Autodesk Fusion 360 part; units mm, degrees
(part 7 of 8)
sketch "Sketch4" plane through (0, 0, 10) normal (0, 0, 1) x (-1, 0, 0) in component "Sun Gear"
  arc A0 (-13.3583, 2.9772) -> (-13.4807, 2.3614) centre (0, 0) ccw
  arc A1 (-14.5708, 1.5395) -> (-13.4807, 2.3614) centre (-14.4657, 2.534) ccw
  line L0 (-14.5708, 1.5395) -> (-14.9519, 1.5798)
  spline S0 degree 5 poles (-14.9519, 1.5798) (-14.9606, 1.5807) (-14.978, 1.5823) (-15.0041, 1.5839) (-15.039, 1.5847) (-15.0828, 1.5837) (-15.1266, 1.5812) (-15.1705, 1.578) (-15.2144, 1.5742) (-15.2583, 1.5701) (-15.3023, 1.5657) (-15.3463, 1.5609) (-15.3903, 1.5554) (-15.4343, 1.5493) (-15.4783, 1.5425) (-15.5224, 1.535) (-15.5664, 1.527) (-15.6104, 1.5186) (-15.6545, 1.5097) (-15.6985, 1.5005) (-15.7425, 1.4909) (-15.7866, 1.4808) (-15.8306, 1.4704) (-15.8746, 1.4595) (-15.9186, 1.4482) (-15.9626, 1.4365) (-16.0065, 1.4244) (-16.0505, 1.4119) (-16.0944, 1.3991) (-16.1383, 1.3859) (-16.1822, 1.3724) (-16.2261, 1.3585) (-16.2699, 1.3443) (-16.3137, 1.3297) (-16.3575, 1.3147) (-16.4013, 1.2995) (-16.4451, 1.2839) (-16.4888, 1.2679) (-16.5324, 1.2517) (-16.5761, 1.2351) (-16.6197, 1.2182) (-16.6633, 1.201) (-16.7068, 1.1835) (-16.7504, 1.1657) (-16.7938, 1.1475) (-16.8373, 1.1291) (-16.8807, 1.1104) (-16.924, 1.0913) (-16.9674, 1.072) (-17.0106, 1.0524) (-17.0539, 1.0325) (-17.0971, 1.0123) (-17.1402, 0.9918) (-17.1833, 0.9711) (-17.2264, 0.95) (-17.2694, 0.9287) (-17.3123, 0.9071) (-17.3552, 0.8852) (-17.3981, 0.863) (-17.4409, 0.8406) (-17.4837, 0.8179) (-17.5264, 0.795) (-17.569, 0.7717) (-17.6116, 0.7482) (-17.6541, 0.7245) (-17.6966, 0.7004) (-17.7391, 0.6762) (-17.7814, 0.6516) (-17.8237, 0.6268) (-17.866, 0.6018) (-17.9082, 0.5765) (-17.9419, 0.556) (-17.9671, 0.5405) (-17.9839, 0.5302) (-17.9923, 0.525) knots 0 0 0 0 0 0 0.01428571 0.02857143 0.04285714 0.05714286 0.07142857 0.08571429 0.1 0.11428571 0.12857143 0.14285714 0.15714286 0.17142857 0.18571429 0.2 0.21428571 0.22857143 0.24285714 0.25714286 0.27142857 0.28571429 0.3 0.31428571 0.32857143 0.34285714 0.35714286 0.37142857 0.38571429 0.4 0.41428571 0.42857143 0.44285714 0.45714286 0.47142857 0.48571429 0.5 0.51428571 0.52857143 0.54285714 0.55714286 0.57142857 0.58571429 0.6 0.61428571 0.62857143 0.64285714 0.65714286 0.67142857 0.68571429 0.7 0.71428571 0.72857143 0.74285714 0.75714286 0.77142857 0.78571429 0.8 0.81428571 0.82857143 0.84285714 0.85714286 0.87142857 0.88571429 0.9 0.91428571 0.92857143 0.94285714 0.95714286 0.97142857 0.98571429 1 1 1 1 1 1
  arc A2 (-17.9923, 0.525) -> (-17.9923, -0.525) centre (0, 0) ccw
  spline S1 degree 5 poles (-17.9923, -0.525) (-17.9839, -0.5302) (-17.9671, -0.5405) (-17.9419, -0.556) (-17.9082, -0.5765) (-17.866, -0.6018) (-17.8237, -0.6268) (-17.7814, -0.6516) (-17.7391, -0.6762) (-17.6966, -0.7004) (-17.6541, -0.7245) (-17.6116, -0.7482) (-17.569, -0.7717) (-17.5264, -0.795) (-17.4837, -0.8179) (-17.4409, -0.8406) (-17.3981, -0.863) (-17.3552, -0.8852) (-17.3123, -0.9071) (-17.2694, -0.9287) (-17.2264, -0.95) (-17.1833, -0.9711) (-17.1402, -0.9918) (-17.0971, -1.0123) (-17.0539, -1.0325) (-17.0106, -1.0524) (-16.9674, -1.072) (-16.924, -1.0913) (-16.8807, -1.1104) (-16.8373, -1.1291) (-16.7938, -1.1475) (-16.7504, -1.1657) (-16.7068, -1.1835) (-16.6633, -1.201) (-16.6197, -1.2182) (-16.5761, -1.2351) (-16.5324, -1.2517) (-16.4888, -1.2679) (-16.4451, -1.2839) (-16.4013, -1.2995) (-16.3575, -1.3147) (-16.3137, -1.3297) (-16.2699, -1.3443) (-16.2261, -1.3585) (-16.1822, -1.3724) (-16.1383, -1.3859) (-16.0944, -1.3991) (-16.0505, -1.4119) (-16.0065, -1.4244) (-15.9626, -1.4365) (-15.9186, -1.4482) (-15.8746, -1.4595) (-15.8306, -1.4704) (-15.7866, -1.4808) (-15.7425, -1.4909) (-15.6985, -1.5005) (-15.6545, -1.5097) (-15.6104, -1.5186) (-15.5664, -1.527) (-15.5224, -1.535) (-15.4783, -1.5425) (-15.4343, -1.5493) (-15.3903, -1.5554) (-15.3463, -1.5609) (-15.3023, -1.5657) (-15.2583, -1.5701) (-15.2144, -1.5742) (-15.1705, -1.578) (-15.1266, -1.5812) (-15.0828, -1.5837) (-15.039, -1.5847) (-15.0041, -1.5839) (-14.978, -1.5823) (-14.9606, -1.5807) (-14.9519, -1.5798) knots -1 -1 -1 -1 -1 -1 -0.98571429 -0.97142857 -0.95714286 -0.94285714 -0.92857143 -0.91428571 -0.9 -0.88571429 -0.87142857 -0.85714286 -0.84285714 -0.82857143 -0.81428571 -0.8 -0.78571429 -0.77142857 -0.75714286 -0.74285714 -0.72857143 -0.71428571 -0.7 -0.68571429 -0.67142857 -0.65714286 -0.64285714 -0.62857143 -0.61428571 -0.6 -0.58571429 -0.57142857 -0.55714286 -0.54285714 -0.52857143 -0.51428571 -0.5 -0.48571429 -0.47142857 -0.45714286 -0.44285714 -0.42857143 -0.41428571 -0.4 -0.38571429 -0.37142857 -0.35714286 -0.34285714 -0.32857143 -0.31428571 -0.3 -0.28571429 -0.27142857 -0.25714286 -0.24285714 -0.22857143 -0.21428571 -0.2 -0.18571429 -0.17142857 -0.15714286 -0.14285714 -0.12857143 -0.11428571 -0.1 -0.08571429 -0.07142857 -0.05714286 -0.04285714 -0.02857143 -0.01428571 0 0 0 0 0 0
  line L1 (-14.9519, -1.5798) -> (-14.5708, -1.5395)
  arc A3 (-13.4807, -2.3614) -> (-14.5708, -1.5395) centre (-14.4657, -2.534) ccw
  arc A4 (-13.4807, -2.3614) -> (-13.3583, -2.9772) centre (0, 0) ccw
  arc A5 (-14.0508, -4.1537) -> (-13.3583, -2.9772) centre (-14.3343, -3.1947) ccw
  line L2 (-14.0508, -4.1537) -> (-14.4183, -4.2623)
  spline S2 degree 5 poles (-14.4183, -4.2623) (-14.4267, -4.2648) (-14.4433, -4.27) (-14.4681, -4.2785) (-14.5007, -4.2912) (-14.5407, -4.3088) (-14.5803, -4.3278) (-14.6196, -4.3477) (-14.6587, -4.3679) (-14.6977, -4.3885) (-14.7367, -4.4094) (-14.7754, -4.4307) (-14.814, -4.4526) (-14.8523, -4.4751) (-14.8904, -4.4982) (-14.9282, -4.522) (-14.9658, -4.5462) (-15.0033, -4.5709) (-15.0406, -4.5959) (-15.0777, -4.6213) (-15.1147, -4.647) (-15.1516, -4.6731) (-15.1882, -4.6996) (-15.2247, -4.7265) (-15.2611, -4.7538) (-15.2972, -4.7814) (-15.3332, -4.8094) (-15.369, -4.8378) (-15.4047, -4.8665) (-15.4402, -4.8954) (-15.4756, -4.9247) (-15.5108, -4.9544) (-15.5459, -4.9843) (-15.5808, -5.0145) (-15.6155, -5.0451) (-15.6501, -5.076) (-15.6846, -5.1071) (-15.7188, -5.1386) (-15.753, -5.1703) (-15.787, -5.2023) (-15.8208, -5.2346) (-15.8545, -5.2672) (-15.888, -5.3) (-15.9214, -5.3331) (-15.9546, -5.3665) (-15.9877, -5.4002) (-16.0206, -5.4341) (-16.0534, -5.4683) (-16.086, -5.5027) (-16.1185, -5.5374) (-16.1508, -5.5723) (-16.183, -5.6075) (-16.215, -5.6429) (-16.2469, -5.6786) (-16.2786, -5.7145) (-16.3102, -5.7507) (-16.3416, -5.7871) (-16.3729, -5.8237) (-16.404, -5.8606) (-16.435, -5.8977) (-16.4658, -5.935) (-16.4965, -5.9726) (-16.527, -6.0104) (-16.5573, -6.0484) (-16.5875, -6.0866) (-16.6176, -6.1251) (-16.6475, -6.1637) (-16.6773, -6.2026) (-16.7068, -6.2417) (-16.7363, -6.2811) (-16.7656, -6.3206) (-16.7889, -6.3524) (-16.8063, -6.3763) (-16.8179, -6.3923) (-16.8237, -6.4003) knots 0 0 0 0 0 0 0.01428571 0.02857143 0.04285714 0.05714286 0.07142857 0.08571429 0.1 0.11428571 0.12857143 0.14285714 0.15714286 0.17142857 0.18571429 0.2 0.21428571 0.22857143 0.24285714 0.25714286 0.27142857 0.28571429 0.3 0.31428571 0.32857143 0.34285714 0.35714286 0.37142857 0.38571429 0.4 0.41428571 0.42857143 0.44285714 0.45714286 0.47142857 0.48571429 0.5 0.51428571 0.52857143 0.54285714 0.55714286 0.57142857 0.58571429 0.6 0.61428571 0.62857143 0.64285714 0.65714286 0.67142857 0.68571429 0.7 0.71428571 0.72857143 0.74285714 0.75714286 0.77142857 0.78571429 0.8 0.81428571 0.82857143 0.84285714 0.85714286 0.87142857 0.88571429 0.9 0.91428571 0.92857143 0.94285714 0.95714286 0.97142857 0.98571429 1 1 1 1 1 1
  arc A6 (-16.8237, -6.4003) -> (-16.4218, -7.3704) centre (0, 0) ccw
  spline S3 degree 5 poles (-16.4218, -7.3704) (-16.4121, -7.372) (-16.3926, -7.3751) (-16.3633, -7.3797) (-16.3244, -7.3857) (-16.2757, -7.393) (-16.2271, -7.4) (-16.1785, -7.4067) (-16.13, -7.4131) (-16.0815, -7.4193) (-16.0331, -7.4253) (-15.9847, -7.4309) (-15.9363, -7.4364) (-15.888, -7.4415) (-15.8398, -7.4464) (-15.7916, -7.451) (-15.7435, -7.4553) (-15.6954, -7.4594) (-15.6474, -7.4632) (-15.5994, -7.4667) (-15.5515, -7.4699) (-15.5037, -7.4729) (-15.4559, -7.4756) (-15.4082, -7.478) (-15.3606, -7.4801) (-15.313, -7.482) (-15.2655, -7.4835) (-15.2181, -7.4848) (-15.1708, -7.4858) (-15.1235, -7.4865) (-15.0763, -7.4869) (-15.0292, -7.487) (-14.9822, -7.4868) (-14.9353, -7.4864) (-14.8884, -7.4856) (-14.8417, -7.4845) (-14.795, -7.4831) (-14.7484, -7.4814) (-14.7019, -7.4794) (-14.6555, -7.4771) (-14.6093, -7.4744) (-14.5631, -7.4715) (-14.517, -7.4682) (-14.4711, -7.4645) (-14.4252, -7.4606) (-14.3795, -7.4563) (-14.3339, -7.4517) (-14.2884, -7.4467) (-14.243, -7.4414) (-14.1977, -7.4358) (-14.1526, -7.4298) (-14.1077, -7.4234) (-14.0628, -7.4166) (-14.0182, -7.4094) (-13.9737, -7.4018) (-13.9293, -7.3938) (-13.8851, -7.3855) (-13.841, -7.3768) (-13.7971, -7.3678) (-13.7534, -7.3583) (-13.7098, -7.3484) (-13.6665, -7.3378) (-13.6235, -7.3266) (-13.5808, -7.3148) (-13.5383, -7.3025) (-13.496, -7.2897) (-13.4539, -7.2767) (-13.4118, -7.2633) (-13.3701, -7.2496) (-13.3286, -7.235) (-13.2878, -7.2192) (-13.2559, -7.2052) (-13.2323, -7.1937) (-13.2168, -7.1855) (-13.2092, -7.1813) knots -1 -1 -1 -1 -1 -1 -0.98571429 -0.97142857 -0.95714286 -0.94285714 -0.92857143 -0.91428571 -0.9 -0.88571429 -0.87142857 -0.85714286 -0.84285714 -0.82857143 -0.81428571 -0.8 -0.78571429 -0.77142857 -0.75714286 -0.74285714 -0.72857143 -0.71428571 -0.7 -0.68571429 -0.67142857 -0.65714286 -0.64285714 -0.62857143 -0.61428571 -0.6 -0.58571429 -0.57142857 -0.55714286 -0.54285714 -0.52857143 -0.51428571 -0.5 -0.48571429 -0.47142857 -0.45714286 -0.44285714 -0.42857143 -0.41428571 -0.4 -0.38571429 -0.37142857 -0.35714286 -0.34285714 -0.32857143 -0.31428571 -0.3 -0.28571429 -0.27142857 -0.25714286 -0.24285714 -0.22857143 -0.21428571 -0.2 -0.18571429 -0.17142857 -0.15714286 -0.14285714 -0.12857143 -0.11428571 -0.1 -0.08571429 -0.07142857 -0.05714286 -0.04285714 -0.02857143 -0.01428571 0 0 0 0 0 0
  line L3 (-13.2092, -7.1813) -> (-12.8725, -6.9983)
  arc A7 (-11.5509, -7.3405) -> (-12.8725, -6.9983) centre (-12.3949, -7.8769) ccw
  arc A8 (-11.5509, -7.3405) -> (-11.2021, -7.8625) centre (0, 0) ccw
  arc A9 (-11.3917, -9.2145) -> (-11.2021, -7.8625) centre (-12.0206, -8.437) ccw
  line L4 (-11.3917, -9.2145) -> (-11.6896, -9.4555)
  spline S4 degree 5 poles (-11.6896, -9.4555) (-11.6964, -9.461) (-11.7099, -9.4722) (-11.7295, -9.4895) (-11.7547, -9.5137) (-11.785, -9.5453) (-11.8142, -9.578) (-11.8429, -9.6114) (-11.8713, -9.6451) (-11.8995, -9.679) (-11.9275, -9.7132) (-11.9552, -9.7478) (-11.9824, -9.7827) (-12.0092, -9.8182) (-12.0355, -9.8541) (-12.0614, -9.8905) (-12.0869, -9.9273) (-12.112, -9.9645) (-12.1369, -10.0019) (-12.1615, -10.0395) (-12.1859, -10.0775) (-12.2099, -10.1157) (-12.2336, -10.1542) (-12.2571, -10.193) (-12.2802, -10.2321) (-12.303, -10.2715) (-12.3255, -10.3111) (-12.3478, -10.351) (-12.3698, -10.3911) (-12.3915, -10.4315) (-12.413, -10.4721) (-12.4342, -10.513) (-12.4551, -10.554) (-12.4758, -10.5953) (-12.4962, -10.6369) (-12.5163, -10.6786) (-12.5362, -10.7206) (-12.5559, -10.7628) (-12.5753, -10.8051) (-12.5944, -10.8477) (-12.6133, -10.8905) (-12.632, -10.9335) (-12.6504, -10.9767) (-12.6686, -11.02) (-12.6865, -11.0636) (-12.7042, -11.1074) (-12.7216, -11.1513) (-12.7388, -11.1954) (-12.7558, -11.2397) (-12.7725, -11.2842) (-12.789, -11.3288) (-12.8053, -11.3736) (-12.8213, -11.4186) (-12.8371, -11.4638) (-12.8526, -11.5091) (-12.868, -11.5546) (-12.8831, -11.6003) (-12.8979, -11.6461) (-12.9126, -11.692) (-12.927, -11.7382) (-12.9412, -11.7845) (-12.9551, -11.8309) (-12.9689, -11.8775) (-12.9824, -11.9242) (-12.9956, -11.9711) (-13.0087, -12.0181) (-13.0215, -12.0653) (-13.0341, -12.1126) (-13.0465, -12.16) (-13.0587, -12.2076) (-13.0706, -12.2554) (-13.08, -12.2937) (-13.0869, -12.3224) (-13.0915, -12.3417) (-13.0937, -12.3513) knots 0 0 0 0 0 0 0.01428571 0.02857143 0.04285714 0.05714286 0.07142857 0.08571429 0.1 0.11428571 0.12857143 0.14285714 0.15714286 0.17142857 0.18571429 0.2 0.21428571 0.22857143 0.24285714 0.25714286 0.27142857 0.28571429 0.3 0.31428571 0.32857143 0.34285714 0.35714286 0.37142857 0.38571429 0.4 0.41428571 0.42857143 0.44285714 0.45714286 0.47142857 0.48571429 0.5 0.51428571 0.52857143 0.54285714 0.55714286 0.57142857 0.58571429 0.6 0.61428571 0.62857143 0.64285714 0.65714286 0.67142857 0.68571429 0.7 0.71428571 0.72857143 0.74285714 0.75714286 0.77142857 0.78571429 0.8 0.81428571 0.82857143 0.84285714 0.85714286 0.87142857 0.88571429 0.9 0.91428571 0.92857143 0.94285714 0.95714286 0.97142857 0.98571429 1 1 1 1 1 1
  arc A10 (-13.0937, -12.3513) -> (-12.3513, -13.0937) centre (0, 0) ccw
  spline S5 degree 5 poles (-12.3513, -13.0937) (-12.3417, -13.0915) (-12.3224, -13.0869) (-12.2937, -13.08) (-12.2554, -13.0706) (-12.2076, -13.0587) (-12.16, -13.0465) (-12.1126, -13.0341) (-12.0653, -13.0215) (-12.0181, -13.0087) (-11.9711, -12.9956) (-11.9242, -12.9824) (-11.8775, -12.9689) (-11.8309, -12.9551) (-11.7845, -12.9412) (-11.7382, -12.927) (-11.692, -12.9126) (-11.6461, -12.8979) (-11.6003, -12.8831) (-11.5546, -12.868) (-11.5091, -12.8526) (-11.4638, -12.8371) (-11.4186, -12.8213) (-11.3736, -12.8053) (-11.3288, -12.789) (-11.2842, -12.7725) (-11.2397, -12.7558) (-11.1954, -12.7388) (-11.1513, -12.7216) (-11.1074, -12.7042) (-11.0636, -12.6865) (-11.02, -12.6686) (-10.9767, -12.6504) (-10.9335, -12.632) (-10.8905, -12.6133) (-10.8477, -12.5944) (-10.8051, -12.5753) (-10.7628, -12.5559) (-10.7206, -12.5362) (-10.6786, -12.5163) (-10.6369, -12.4962) (-10.5953, -12.4758) (-10.554, -12.4551) (-10.513, -12.4342) (-10.4721, -12.413) (-10.4315, -12.3915) (-10.3911, -12.3698) (-10.351, -12.3478) (-10.3111, -12.3255) (-10.2715, -12.303) (-10.2321, -12.2802) (-10.193, -12.2571) (-10.1542, -12.2336) (-10.1157, -12.2099) (-10.0775, -12.1859) (-10.0395, -12.1615) (-10.0019, -12.1369) (-9.9645, -12.112) (-9.9273, -12.0869) (-9.8905, -12.0614) (-9.8541, -12.0355) (-9.8182, -12.0092) (-9.7827, -11.9824) (-9.7478, -11.9552) (-9.7132, -11.9275) (-9.679, -11.8995) (-9.6451, -11.8713) (-9.6114, -11.8429) (-9.578, -11.8142) (-9.5453, -11.785) (-9.5137, -11.7547) (-9.4895, -11.7295) (-9.4722, -11.7099) (-9.461, -11.6964) (-9.4555, -11.6896) knots -1 -1 -1 -1 -1 -1 -0.98571429 -0.97142857 -0.95714286 -0.94285714 -0.92857143 -0.91428571 -0.9 -0.88571429 -0.87142857 -0.85714286 -0.84285714 -0.82857143 -0.81428571 -0.8 -0.78571429 -0.77142857 -0.75714286 -0.74285714 -0.72857143 -0.71428571 -0.7 -0.68571429 -0.67142857 -0.65714286 -0.64285714 -0.62857143 -0.61428571 -0.6 -0.58571429 -0.57142857 -0.55714286 -0.54285714 -0.52857143 -0.51428571 -0.5 -0.48571429 -0.47142857 -0.45714286 -0.44285714 -0.42857143 -0.41428571 -0.4 -0.38571429 -0.37142857 -0.35714286 -0.34285714 -0.32857143 -0.31428571 -0.3 -0.28571429 -0.27142857 -0.25714286 -0.24285714 -0.22857143 -0.21428571 -0.2 -0.18571429 -0.17142857 -0.15714286 -0.14285714 -0.12857143 -0.11428571 -0.1 -0.08571429 -0.07142857 -0.05714286 -0.04285714 -0.02857143 -0.01428571 0 0 0 0 0 0
  line L5 (-9.4555, -11.6896) -> (-9.2145, -11.3917)
  arc A11 (-7.8625, -11.2021) -> (-9.2145, -11.3917) centre (-8.437, -12.0206) ccw
  arc A12 (-7.8625, -11.2021) -> (-7.3405, -11.5509) centre (0, 0) ccw
  arc A13 (-6.9983, -12.8725) -> (-7.3405, -11.5509) centre (-7.8769, -12.3949) ccw
  line L6 (-6.9983, -12.8725) -> (-7.1813, -13.2092)
  spline S6 degree 5 poles (-7.1813, -13.2092) (-7.1855, -13.2168) (-7.1937, -13.2323) (-7.2052, -13.2559) (-7.2192, -13.2878) (-7.235, -13.3286) (-7.2496, -13.3701) (-7.2633, -13.4118) (-7.2767, -13.4539) (-7.2897, -13.496) (-7.3025, -13.5383) (-7.3148, -13.5808) (-7.3266, -13.6235) (-7.3378, -13.6665) (-7.3484, -13.7098) (-7.3583, -13.7534) (-7.3678, -13.7971) (-7.3768, -13.841) (-7.3855, -13.8851) (-7.3938, -13.9293) (-7.4018, -13.9737) (-7.4094, -14.0182) (-7.4166, -14.0628) (-7.4234, -14.1077) (-7.4298, -14.1526) (-7.4358, -14.1977) (-7.4414, -14.243) (-7.4467, -14.2884) (-7.4517, -14.3339) (-7.4563, -14.3795) (-7.4606, -14.4252) (-7.4645, -14.4711) (-7.4682, -14.517) (-7.4715, -14.5631) (-7.4744, -14.6093) (-7.4771, -14.6555) (-7.4794, -14.7019) (-7.4814, -14.7484) (-7.4831, -14.795) (-7.4845, -14.8417) (-7.4856, -14.8884) (-7.4864, -14.9353) (-7.4868, -14.9822) (-7.487, -15.0292) (-7.4869, -15.0763) (-7.4865, -15.1235) (-7.4858, -15.1708) (-7.4848, -15.2181) (-7.4835, -15.2655) (-7.482, -15.313) (-7.4801, -15.3606) (-7.478, -15.4082) (-7.4756, -15.4559) (-7.4729, -15.5037) (-7.4699, -15.5515) (-7.4667, -15.5994) (-7.4632, -15.6474) (-7.4594, -15.6954) (-7.4553, -15.7435) (-7.451, -15.7916) (-7.4464, -15.8398) (-7.4415, -15.888) (-7.4364, -15.9363) (-7.4309, -15.9847) (-7.4253, -16.0331) (-7.4193, -16.0815) (-7.4131, -16.13) (-7.4067, -16.1785) (-7.4, -16.2271) (-7.393, -16.2757) (-7.3857, -16.3244) (-7.3797, -16.3633) (-7.3751, -16.3926) (-7.372, -16.4121) (-7.3704, -16.4218) knots 0 0 0 0 0 0 0.01428571 0.02857143 0.04285714 0.05714286 0.07142857 0.08571429 0.1 0.11428571 0.12857143 0.14285714 0.15714286 0.17142857 0.18571429 0.2 0.21428571 0.22857143 0.24285714 0.25714286 0.27142857 0.28571429 0.3 0.31428571 0.32857143 0.34285714 0.35714286 0.37142857 0.38571429 0.4 0.41428571 0.42857143 0.44285714 0.45714286 0.47142857 0.48571429 0.5 0.51428571 0.52857143 0.54285714 0.55714286 0.57142857 0.58571429 0.6 0.61428571 0.62857143 0.64285714 0.65714286 0.67142857 0.68571429 0.7 0.71428571 0.72857143 0.74285714 0.75714286 0.77142857 0.78571429 0.8 0.81428571 0.82857143 0.84285714 0.85714286 0.87142857 0.88571429 0.9 0.91428571 0.92857143 0.94285714 0.95714286 0.97142857 0.98571429 1 1 1 1 1 1
  arc A14 (-7.3704, -16.4218) -> (-6.4003, -16.8237) centre (0, 0) ccw
  spline S7 degree 5 poles (-6.4003, -16.8237) (-6.3923, -16.8179) (-6.3763, -16.8063) (-6.3524, -16.7889) (-6.3206, -16.7656) (-6.2811, -16.7363) (-6.2417, -16.7068) (-6.2026, -16.6773) (-6.1637, -16.6475) (-6.1251, -16.6176) (-6.0866, -16.5875) (-6.0484, -16.5573) (-6.0104, -16.527) (-5.9726, -16.4965) (-5.935, -16.4658) (-5.8977, -16.435) (-5.8606, -16.404) (-5.8237, -16.3729) (-5.7871, -16.3416) (-5.7507, -16.3102) (-5.7145, -16.2786) (-5.6786, -16.2469) (-5.6429, -16.215) (-5.6075, -16.183) (-5.5723, -16.1508) (-5.5374, -16.1185) (-5.5027, -16.086) (-5.4683, -16.0534) (-5.4341, -16.0206) (-5.4002, -15.9877) (-5.3665, -15.9546) (-5.3331, -15.9214) (-5.3, -15.888) (-5.2672, -15.8545) (-5.2346, -15.8208) (-5.2023, -15.787) (-5.1703, -15.753) (-5.1386, -15.7188) (-5.1071, -15.6846) (-5.076, -15.6501) (-5.0451, -15.6155) (-5.0145, -15.5808) (-4.9843, -15.5459) (-4.9544, -15.5108) (-4.9247, -15.4756) (-4.8954, -15.4402) (-4.8665, -15.4047) (-4.8378, -15.369) (-4.8094, -15.3332) (-4.7814, -15.2972) (-4.7538, -15.2611) (-4.7265, -15.2247) (-4.6996, -15.1882) (-4.6731, -15.1516) (-4.647, -15.1147) (-4.6213, -15.0777) (-4.5959, -15.0406) (-4.5709, -15.0033) (-4.5462, -14.9658) (-4.522, -14.9282) (-4.4982, -14.8904) (-4.4751, -14.8523) (-4.4526, -14.814) (-4.4307, -14.7754) (-4.4094, -14.7367) (-4.3885, -14.6977) (-4.3679, -14.6587) (-4.3477, -14.6196) (-4.3278, -14.5803) (-4.3088, -14.5407) (-4.2912, -14.5007) (-4.2785, -14.4681) (-4.27, -14.4433) (-4.2648, -14.4267) (-4.2623, -14.4183) knots -1 -1 -1 -1 -1 -1 -0.98571429 -0.97142857 -0.95714286 -0.94285714 -0.92857143 -0.91428571 -0.9 -0.88571429 -0.87142857 -0.85714286 -0.84285714 -0.82857143 -0.81428571 -0.8 -0.78571429 -0.77142857 -0.75714286 -0.74285714 -0.72857143 -0.71428571 -0.7 -0.68571429 -0.67142857 -0.65714286 -0.64285714 -0.62857143 -0.61428571 -0.6 -0.58571429 -0.57142857 -0.55714286 -0.54285714 -0.52857143 -0.51428571 -0.5 -0.48571429 -0.47142857 -0.45714286 -0.44285714 -0.42857143 -0.41428571 -0.4 -0.38571429 -0.37142857 -0.35714286 -0.34285714 -0.32857143 -0.31428571 -0.3 -0.28571429 -0.27142857 -0.25714286 -0.24285714 -0.22857143 -0.21428571 -0.2 -0.18571429 -0.17142857 -0.15714286 -0.14285714 -0.12857143 -0.11428571 -0.1 -0.08571429 -0.07142857 -0.05714286 -0.04285714 -0.02857143 -0.01428571 0 0 0 0 0 0
  line L7 (-4.2623, -14.4183) -> (-4.1537, -14.0508)
  arc A15 (-2.9772, -13.3583) -> (-4.1537, -14.0508) centre (-3.1947, -14.3343) ccw
  arc A16 (-2.9772, -13.3583) -> (-2.3614, -13.4807) centre (0, 0) ccw
  arc A17 (-1.5395, -14.5708) -> (-2.3614, -13.4807) centre (-2.534, -14.4657) ccw
  line L8 (-1.5395, -14.5708) -> (-1.5798, -14.9519)
  spline S8 degree 5 poles (-1.5798, -14.9519) (-1.5807, -14.9606) (-1.5823, -14.978) (-1.5839, -15.0041) (-1.5847, -15.039) (-1.5837, -15.0828) (-1.5812, -15.1266) (-1.578, -15.1705) (-1.5742, -15.2144) (-1.5701, -15.2583) (-1.5657, -15.3023) (-1.5609, -15.3463) (-1.5554, -15.3903) (-1.5493, -15.4343) (-1.5425, -15.4783) (-1.535, -15.5224) (-1.527, -15.5664) (-1.5186, -15.6104) (-1.5097, -15.6545) (-1.5005, -15.6985) (-1.4909, -15.7425) (-1.4808, -15.7866) (-1.4704, -15.8306) (-1.4595, -15.8746) (-1.4482, -15.9186) (-1.4365, -15.9626) (-1.4244, -16.0065) (-1.4119, -16.0505) (-1.3991, -16.0944) (-1.3859, -16.1383) (-1.3724, -16.1822) (-1.3585, -16.2261) (-1.3443, -16.2699) (-1.3297, -16.3137) (-1.3147, -16.3575) (-1.2995, -16.4013) (-1.2839, -16.4451) (-1.2679, -16.4888) (-1.2517, -16.5324) (-1.2351, -16.5761) (-1.2182, -16.6197) (-1.201, -16.6633) (-1.1835, -16.7068) (-1.1657, -16.7504) (-1.1475, -16.7938) (-1.1291, -16.8373) (-1.1104, -16.8807) (-1.0913, -16.924) (-1.072, -16.9674) (-1.0524, -17.0106) (-1.0325, -17.0539) (-1.0123, -17.0971) (-0.9918, -17.1402) (-0.9711, -17.1833) (-0.95, -17.2264) (-0.9287, -17.2694) (-0.9071, -17.3123) (-0.8852, -17.3552) (-0.863, -17.3981) (-0.8406, -17.4409) (-0.8179, -17.4837) (-0.795, -17.5264) (-0.7717, -17.569) (-0.7482, -17.6116) (-0.7245, -17.6541) (-0.7004, -17.6966) (-0.6762, -17.7391) (-0.6516, -17.7814) (-0.6268, -17.8237) (-0.6018, -17.866) (-0.5765, -17.9082) (-0.556, -17.9419) (-0.5405, -17.9671) (-0.5302, -17.9839) (-0.525, -17.9923) knots 0 0 0 0 0 0 0.01428571 0.02857143 0.04285714 0.05714286 0.07142857 0.08571429 0.1 0.11428571 0.12857143 0.14285714 0.15714286 0.17142857 0.18571429 0.2 0.21428571 0.22857143 0.24285714 0.25714286 0.27142857 0.28571429 0.3 0.31428571 0.32857143 0.34285714 0.35714286 0.37142857 0.38571429 0.4 0.41428571 0.42857143 0.44285714 0.45714286 0.47142857 0.48571429 0.5 0.51428571 0.52857143 0.54285714 0.55714286 0.57142857 0.58571429 0.6 0.61428571 0.62857143 0.64285714 0.65714286 0.67142857 0.68571429 0.7 0.71428571 0.72857143 0.74285714 0.75714286 0.77142857 0.78571429 0.8 0.81428571 0.82857143 0.84285714 0.85714286 0.87142857 0.88571429 0.9 0.91428571 0.92857143 0.94285714 0.95714286 0.97142857 0.98571429 1 1 1 1 1 1
  arc A18 (-0.525, -17.9923) -> (0.525, -17.9923) centre (0, 0) ccw
  spline S9 degree 5 poles (0.525, -17.9923) (0.5302, -17.9839) (0.5405, -17.9671) (0.556, -17.9419) (0.5765, -17.9082) (0.6018, -17.866) (0.6268, -17.8237) (0.6516, -17.7814) (0.6762, -17.7391) (0.7004, -17.6966) (0.7245, -17.6541) (0.7482, -17.6116) (0.7717, -17.569) (0.795, -17.5264) (0.8179, -17.4837) (0.8406, -17.4409) (0.863, -17.3981) (0.8852, -17.3552) (0.9071, -17.3123) (0.9287, -17.2694) (0.95, -17.2264) (0.9711, -17.1833) (0.9918, -17.1402) (1.0123, -17.0971) (1.0325, -17.0539) (1.0524, -17.0106) (1.072, -16.9674) (1.0913, -16.924) (1.1104, -16.8807) (1.1291, -16.8373) (1.1475, -16.7938) (1.1657, -16.7504) (1.1835, -16.7068) (1.201, -16.6633) (1.2182, -16.6197) (1.2351, -16.5761) (1.2517, -16.5324) (1.2679, -16.4888) (1.2839, -16.4451) (1.2995, -16.4013) (1.3147, -16.3575) (1.3297, -16.3137) (1.3443, -16.2699) (1.3585, -16.2261) (1.3724, -16.1822) (1.3859, -16.1383) (1.3991, -16.0944) (1.4119, -16.0505) (1.4244, -16.0065) (1.4365, -15.9626) (1.4482, -15.9186) (1.4595, -15.8746) (1.4704, -15.8306) (1.4808, -15.7866) (1.4909, -15.7425) (1.5005, -15.6985) (1.5097, -15.6545) (1.5186, -15.6104) (1.527, -15.5664) (1.535, -15.5224) (1.5425, -15.4783) (1.5493, -15.4343) (1.5554, -15.3903) (1.5609, -15.3463) (1.5657, -15.3023) (1.5701, -15.2583) (1.5742, -15.2144) (1.578, -15.1705) (1.5812, -15.1266) (1.5837, -15.0828) (1.5847, -15.039) (1.5839, -15.0041) (1.5823, -14.978) (1.5807, -14.9606) (1.5798, -14.9519) knots -1 -1 -1 -1 -1 -1 -0.98571429 -0.97142857 -0.95714286 -0.94285714 -0.92857143 -0.91428571 -0.9 -0.88571429 -0.87142857 -0.85714286 -0.84285714 -0.82857143 -0.81428571 -0.8 -0.78571429 -0.77142857 -0.75714286 -0.74285714 -0.72857143 -0.71428571 -0.7 -0.68571429 -0.67142857 -0.65714286 -0.64285714 -0.62857143 -0.61428571 -0.6 -0.58571429 -0.57142857 -0.55714286 -0.54285714 -0.52857143 -0.51428571 -0.5 -0.48571429 -0.47142857 -0.45714286 -0.44285714 -0.42857143 -0.41428571 -0.4 -0.38571429 -0.37142857 -0.35714286 -0.34285714 -0.32857143 -0.31428571 -0.3 -0.28571429 -0.27142857 -0.25714286 -0.24285714 -0.22857143 -0.21428571 -0.2 -0.18571429 -0.17142857 -0.15714286 -0.14285714 -0.12857143 -0.11428571 -0.1 -0.08571429 -0.07142857 -0.05714286 -0.04285714 -0.02857143 -0.01428571 0 0 0 0 0 0
  line L9 (1.5798, -14.9519) -> (1.5395, -14.5708)
  arc A19 (2.3614, -13.4807) -> (1.5395, -14.5708) centre (2.534, -14.4657) ccw
  arc A20 (2.3614, -13.4807) -> (2.9772, -13.3583) centre (0, 0) ccw
  arc A21 (4.1537, -14.0508) -> (2.9772, -13.3583) centre (3.1947, -14.3343) ccw
  line L10 (4.1537, -14.0508) -> (4.2623, -14.4183)
  spline S10 degree 5 poles (4.2623, -14.4183) (4.2648, -14.4267) (4.27, -14.4433) (4.2785, -14.4681) (4.2912, -14.5007) (4.3088, -14.5407) (4.3278, -14.5803) (4.3477, -14.6196) (4.3679, -14.6587) (4.3885, -14.6977) (4.4094, -14.7367) (4.4307, -14.7754) (4.4526, -14.814) (4.4751, -14.8523) (4.4982, -14.8904) (4.522, -14.9282) (4.5462, -14.9658) (4.5709, -15.0033) (4.5959, -15.0406) (4.6213, -15.0777) (4.647, -15.1147) (4.6731, -15.1516) (4.6996, -15.1882) (4.7265, -15.2247) (4.7538, -15.2611) (4.7814, -15.2972) (4.8094, -15.3332) (4.8378, -15.369) (4.8665, -15.4047) (4.8954, -15.4402) (4.9247, -15.4756) (4.9544, -15.5108) (4.9843, -15.5459) (5.0145, -15.5808) (5.0451, -15.6155) (5.076, -15.6501) (5.1071, -15.6846) (5.1386, -15.7188) (5.1703, -15.753) (5.2023, -15.787) (5.2346, -15.8208) (5.2672, -15.8545) (5.3, -15.888) (5.3331, -15.9214) (5.3665, -15.9546) (5.4002, -15.9877) (5.4341, -16.0206) (5.4683, -16.0534) (5.5027, -16.086) (5.5374, -16.1185) (5.5723, -16.1508) (5.6075, -16.183) (5.6429, -16.215) (5.6786, -16.2469) (5.7145, -16.2786) (5.7507, -16.3102) (5.7871, -16.3416) (5.8237, -16.3729) (5.8606, -16.404) (5.8977, -16.435) (5.935, -16.4658) (5.9726, -16.4965) (6.0104, -16.527) (6.0484, -16.5573) (6.0866, -16.5875) (6.1251, -16.6176) (6.1637, -16.6475) (6.2026, -16.6773) (6.2417, -16.7068) (6.2811, -16.7363) (6.3206, -16.7656) (6.3524, -16.7889) (6.3763, -16.8063) (6.3923, -16.8179) (6.4003, -16.8237) knots 0 0 0 0 0 0 0.01428571 0.02857143 0.04285714 0.05714286 0.07142857 0.08571429 0.1 0.11428571 0.12857143 0.14285714 0.15714286 0.17142857 0.18571429 0.2 0.21428571 0.22857143 0.24285714 0.25714286 0.27142857 0.28571429 0.3 0.31428571 0.32857143 0.34285714 0.35714286 0.37142857 0.38571429 0.4 0.41428571 0.42857143 0.44285714 0.45714286 0.47142857 0.48571429 0.5 0.51428571 0.52857143 0.54285714 0.55714286 0.57142857 0.58571429 0.6 0.61428571 0.62857143 0.64285714 0.65714286 0.67142857 0.68571429 0.7 0.71428571 0.72857143 0.74285714 0.75714286 0.77142857 0.78571429 0.8 0.81428571 0.82857143 0.84285714 0.85714286 0.87142857 0.88571429 0.9 0.91428571 0.92857143 0.94285714 0.95714286 0.97142857 0.98571429 1 1 1 1 1 1
  arc A22 (6.4003, -16.8237) -> (7.3704, -16.4218) centre (0, 0) ccw
  spline S11 degree 5 poles (7.3704, -16.4218) (7.372, -16.4121) (7.3751, -16.3926) (7.3797, -16.3633) (7.3857, -16.3244) (7.393, -16.2757) (7.4, -16.2271) (7.4067, -16.1785) (7.4131, -16.13) (7.4193, -16.0815) (7.4253, -16.0331) (7.4309, -15.9847) (7.4364, -15.9363) (7.4415, -15.888) (7.4464, -15.8398) (7.451, -15.7916) (7.4553, -15.7435) (7.4594, -15.6954) (7.4632, -15.6474) (7.4667, -15.5994) (7.4699, -15.5515) (7.4729, -15.5037) (7.4756, -15.4559) (7.478, -15.4082) (7.4801, -15.3606) (7.482, -15.313) (7.4835, -15.2655) (7.4848, -15.2181) (7.4858, -15.1708) (7.4865, -15.1235) (7.4869, -15.0763) (7.487, -15.0292) (7.4868, -14.9822) (7.4864, -14.9353) (7.4856, -14.8884) (7.4845, -14.8417) (7.4831, -14.795) (7.4814, -14.7484) (7.4794, -14.7019) (7.4771, -14.6555) (7.4744, -14.6093) (7.4715, -14.5631) (7.4682, -14.517) (7.4645, -14.4711) (7.4606, -14.4252) (7.4563, -14.3795) (7.4517, -14.3339) (7.4467, -14.2884) (7.4414, -14.243) (7.4358, -14.1977) (7.4298, -14.1526) (7.4234, -14.1077) (7.4166, -14.0628) (7.4094, -14.0182) (7.4018, -13.9737) (7.3938, -13.9293) (7.3855, -13.8851) (7.3768, -13.841) (7.3678, -13.7971) (7.3583, -13.7534) (7.3484, -13.7098) (7.3378, -13.6665) (7.3266, -13.6235) (7.3148, -13.5808) (7.3025, -13.5383) (7.2897, -13.496) (7.2767, -13.4539) (7.2633, -13.4118) (7.2496, -13.3701) (7.235, -13.3286) (7.2192, -13.2878) (7.2052, -13.2559) (7.1937, -13.2323) (7.1855, -13.2168) (7.1813, -13.2092) knots -1 -1 -1 -1 -1 -1 -0.98571429 -0.97142857 -0.95714286 -0.94285714 -0.92857143 -0.91428571 -0.9 -0.88571429 -0.87142857 -0.85714286 -0.84285714 -0.82857143 -0.81428571 -0.8 -0.78571429 -0.77142857 -0.75714286 -0.74285714 -0.72857143 -0.71428571 -0.7 -0.68571429 -0.67142857 -0.65714286 -0.64285714 -0.62857143 -0.61428571 -0.6 -0.58571429 -0.57142857 -0.55714286 -0.54285714 -0.52857143 -0.51428571 -0.5 -0.48571429 -0.47142857 -0.45714286 -0.44285714 -0.42857143 -0.41428571 -0.4 -0.38571429 -0.37142857 -0.35714286 -0.34285714 -0.32857143 -0.31428571 -0.3 -0.28571429 -0.27142857 -0.25714286 -0.24285714 -0.22857143 -0.21428571 -0.2 -0.18571429 -0.17142857 -0.15714286 -0.14285714 -0.12857143 -0.11428571 -0.1 -0.08571429 -0.07142857 -0.05714286 -0.04285714 -0.02857143 -0.01428571 0 0 0 0 0 0
  line L11 (7.1813, -13.2092) -> (6.9983, -12.8725)
  arc A23 (7.3405, -11.5509) -> (6.9983, -12.8725) centre (7.8769, -12.3949) ccw
  arc A24 (7.3405, -11.5509) -> (7.8625, -11.2021) centre (0, 0) ccw
  arc A25 (9.2145, -11.3917) -> (7.8625, -11.2021) centre (8.437, -12.0206) ccw
  line L12 (9.2145, -11.3917) -> (9.4555, -11.6896)
  spline S12 degree 5 poles (9.4555, -11.6896) (9.461, -11.6964) (9.4722, -11.7099) (9.4895, -11.7295) (9.5137, -11.7547) (9.5453, -11.785) (9.578, -11.8142) (9.6114, -11.8429) (9.6451, -11.8713) (9.679, -11.8995) (9.7132, -11.9275) (9.7478, -11.9552) (9.7827, -11.9824) (9.8182, -12.0092) (9.8541, -12.0355) (9.8905, -12.0614) (9.9273, -12.0869) (9.9645, -12.112) (10.0019, -12.1369) (10.0395, -12.1615) (10.0775, -12.1859) (10.1157, -12.2099) (10.1542, -12.2336) (10.193, -12.2571) (10.2321, -12.2802) (10.2715, -12.303) (10.3111, -12.3255) (10.351, -12.3478) (10.3911, -12.3698) (10.4315, -12.3915) (10.4721, -12.413) (10.513, -12.4342) (10.554, -12.4551) (10.5953, -12.4758) (10.6369, -12.4962) (10.6786, -12.5163) (10.7206, -12.5362) (10.7628, -12.5559) (10.8051, -12.5753) (10.8477, -12.5944) (10.8905, -12.6133) (10.9335, -12.632) (10.9767, -12.6504) (11.02, -12.6686) (11.0636, -12.6865) (11.1074, -12.7042) (11.1513, -12.7216) (11.1954, -12.7388) (11.2397, -12.7558) (11.2842, -12.7725) (11.3288, -12.789) (11.3736, -12.8053) (11.4186, -12.8213) (11.4638, -12.8371) (11.5091, -12.8526) (11.5546, -12.868) (11.6003, -12.8831) (11.6461, -12.8979) (11.692, -12.9126) (11.7382, -12.927) (11.7845, -12.9412) (11.8309, -12.9551) (11.8775, -12.9689) (11.9242, -12.9824) (11.9711, -12.9956) (12.0181, -13.0087) (12.0653, -13.0215) (12.1126, -13.0341) (12.16, -13.0465) (12.2076, -13.0587) (12.2554, -13.0706) (12.2937, -13.08) (12.3224, -13.0869) (12.3417, -13.0915) (12.3513, -13.0937) knots 0 0 0 0 0 0 0.01428571 0.02857143 0.04285714 0.05714286 0.07142857 0.08571429 0.1 0.11428571 0.12857143 0.14285714 0.15714286 0.17142857 0.18571429 0.2 0.21428571 0.22857143 0.24285714 0.25714286 0.27142857 0.28571429 0.3 0.31428571 0.32857143 0.34285714 0.35714286 0.37142857 0.38571429 0.4 0.41428571 0.42857143 0.44285714 0.45714286 0.47142857 0.48571429 0.5 0.51428571 0.52857143 0.54285714 0.55714286 0.57142857 0.58571429 0.6 0.61428571 0.62857143 0.64285714 0.65714286 0.67142857 0.68571429 0.7 0.71428571 0.72857143 0.74285714 0.75714286 0.77142857 0.78571429 0.8 0.81428571 0.82857143 0.84285714 0.85714286 0.87142857 0.88571429 0.9 0.91428571 0.92857143 0.94285714 0.95714286 0.97142857 0.98571429 1 1 1 1 1 1
  arc A26 (12.3513, -13.0937) -> (13.0937, -12.3513) centre (0, 0) ccw
  spline S13 degree 5 poles (13.0937, -12.3513) (13.0915, -12.3417) (13.0869, -12.3224) (13.08, -12.2937) (13.0706, -12.2554) (13.0587, -12.2076) (13.0465, -12.16) (13.0341, -12.1126) (13.0215, -12.0653) (13.0087, -12.0181) (12.9956, -11.9711) (12.9824, -11.9242) (12.9689, -11.8775) (12.9551, -11.8309) (12.9412, -11.7845) (12.927, -11.7382) (12.9126, -11.692) (12.8979, -11.6461) (12.8831, -11.6003) (12.868, -11.5546) (12.8526, -11.5091) (12.8371, -11.4638) (12.8213, -11.4186) (12.8053, -11.3736) (12.789, -11.3288) (12.7725, -11.2842) (12.7558, -11.2397) (12.7388, -11.1954) (12.7216, -11.1513) (12.7042, -11.1074) (12.6865, -11.0636) (12.6686, -11.02) (12.6504, -10.9767) (12.632, -10.9335) (12.6133, -10.8905) (12.5944, -10.8477) (12.5753, -10.8051) (12.5559, -10.7628) (12.5362, -10.7206) (12.5163, -10.6786) (12.4962, -10.6369) (12.4758, -10.5953) (12.4551, -10.554) (12.4342, -10.513) (12.413, -10.4721) (12.3915, -10.4315) (12.3698, -10.3911) (12.3478, -10.351) (12.3255, -10.3111) (12.303, -10.2715) (12.2802, -10.2321) (12.2571, -10.193) (12.2336, -10.1542) (12.2099, -10.1157) (12.1859, -10.0775) (12.1615, -10.0395) (12.1369, -10.0019) (12.112, -9.9645) (12.0869, -9.9273) (12.0614, -9.8905) (12.0355, -9.8541) (12.0092, -9.8182) (11.9824, -9.7827) (11.9552, -9.7478) (11.9275, -9.7132) (11.8995, -9.679) (11.8713, -9.6451) (11.8429, -9.6114) (11.8142, -9.578) (11.785, -9.5453) (11.7547, -9.5137) (11.7295, -9.4895) (11.7099, -9.4722) (11.6964, -9.461) (11.6896, -9.4555) knots -1 -1 -1 -1 -1 -1 -0.98571429 -0.97142857 -0.95714286 -0.94285714 -0.92857143 -0.91428571 -0.9 -0.88571429 -0.87142857 -0.85714286 -0.84285714 -0.82857143 -0.81428571 -0.8 -0.78571429 -0.77142857 -0.75714286 -0.74285714 -0.72857143 -0.71428571 -0.7 -0.68571429 -0.67142857 -0.65714286 -0.64285714 -0.62857143 -0.61428571 -0.6 -0.58571429 -0.57142857 -0.55714286 -0.54285714 -0.52857143 -0.51428571 -0.5 -0.48571429 -0.47142857 -0.45714286 -0.44285714 -0.42857143 -0.41428571 -0.4 -0.38571429 -0.37142857 -0.35714286 -0.34285714 -0.32857143 -0.31428571 -0.3 -0.28571429 -0.27142857 -0.25714286 -0.24285714 -0.22857143 -0.21428571 -0.2 -0.18571429 -0.17142857 -0.15714286 -0.14285714 -0.12857143 -0.11428571 -0.1 -0.08571429 -0.07142857 -0.05714286 -0.04285714 -0.02857143 -0.01428571 0 0 0 0 0 0
  line L13 (11.6896, -9.4555) -> (11.3917, -9.2145)
  arc A27 (11.2021, -7.8625) -> (11.3917, -9.2145) centre (12.0206, -8.437) ccw
  arc A28 (11.2021, -7.8625) -> (11.5509, -7.3405) centre (0, 0) ccw
  arc A29 (12.8725, -6.9983) -> (11.5509, -7.3405) centre (12.3949, -7.8769) ccw
  line L14 (12.8725, -6.9983) -> (13.2092, -7.1813)
  spline S14 degree 5 poles (13.2092, -7.1813) (13.2168, -7.1855) (13.2323, -7.1937) (13.2559, -7.2052) (13.2878, -7.2192) (13.3286, -7.235) (13.3701, -7.2496) (13.4118, -7.2633) (13.4539, -7.2767) (13.496, -7.2897) (13.5383, -7.3025) (13.5808, -7.3148) (13.6235, -7.3266) (13.6665, -7.3378) (13.7098, -7.3484) (13.7534, -7.3583) (13.7971, -7.3678) (13.841, -7.3768) (13.8851, -7.3855) (13.9293, -7.3938) (13.9737, -7.4018) (14.0182, -7.4094) (14.0628, -7.4166) (14.1077, -7.4234) (14.1526, -7.4298) (14.1977, -7.4358) (14.243, -7.4414) (14.2884, -7.4467) (14.3339, -7.4517) (14.3795, -7.4563) (14.4252, -7.4606) (14.4711, -7.4645) (14.517, -7.4682) (14.5631, -7.4715) (14.6093, -7.4744) (14.6555, -7.4771) (14.7019, -7.4794) (14.7484, -7.4814) (14.795, -7.4831) (14.8417, -7.4845) (14.8884, -7.4856) (14.9353, -7.4864) (14.9822, -7.4868) (15.0292, -7.487) (15.0763, -7.4869) (15.1235, -7.4865) (15.1708, -7.4858) (15.2181, -7.4848) (15.2655, -7.4835) (15.313, -7.482) (15.3606, -7.4801) (15.4082, -7.478) (15.4559, -7.4756) (15.5037, -7.4729) (15.5515, -7.4699) (15.5994, -7.4667) (15.6474, -7.4632) (15.6954, -7.4594) (15.7435, -7.4553) (15.7916, -7.451) (15.8398, -7.4464) (15.888, -7.4415) (15.9363, -7.4364) (15.9847, -7.4309) (16.0331, -7.4253) (16.0815, -7.4193) (16.13, -7.4131) (16.1785, -7.4067) (16.2271, -7.4) (16.2757, -7.393) (16.3244, -7.3857) (16.3633, -7.3797) (16.3926, -7.3751) (16.4121, -7.372) (16.4218, -7.3704) knots 0 0 0 0 0 0 0.01428571 0.02857143 0.04285714 0.05714286 0.07142857 0.08571429 0.1 0.11428571 0.12857143 0.14285714 0.15714286 0.17142857 0.18571429 0.2 0.21428571 0.22857143 0.24285714 0.25714286 0.27142857 0.28571429 0.3 0.31428571 0.32857143 0.34285714 0.35714286 0.37142857 0.38571429 0.4 0.41428571 0.42857143 0.44285714 0.45714286 0.47142857 0.48571429 0.5 0.51428571 0.52857143 0.54285714 0.55714286 0.57142857 0.58571429 0.6 0.61428571 0.62857143 0.64285714 0.65714286 0.67142857 0.68571429 0.7 0.71428571 0.72857143 0.74285714 0.75714286 0.77142857 0.78571429 0.8 0.81428571 0.82857143 0.84285714 0.85714286 0.87142857 0.88571429 0.9 0.91428571 0.92857143 0.94285714 0.95714286 0.97142857 0.98571429 1 1 1 1 1 1
  arc A30 (16.4218, -7.3704) -> (16.8237, -6.4003) centre (0, 0) ccw
  spline S15 degree 5 poles (16.8237, -6.4003) (16.8179, -6.3923) (16.8063, -6.3763) (16.7889, -6.3524) (16.7656, -6.3206) (16.7363, -6.2811) (16.7068, -6.2417) (16.6773, -6.2026) (16.6475, -6.1637) (16.6176, -6.1251) (16.5875, -6.0866) (16.5573, -6.0484) (16.527, -6.0104) (16.4965, -5.9726) (16.4658, -5.935) (16.435, -5.8977) (16.404, -5.8606) (16.3729, -5.8237) (16.3416, -5.7871) (16.3102, -5.7507) (16.2786, -5.7145) (16.2469, -5.6786) (16.215, -5.6429) (16.183, -5.6075) (16.1508, -5.5723) (16.1185, -5.5374) (16.086, -5.5027) (16.0534, -5.4683) (16.0206, -5.4341) (15.9877, -5.4002) (15.9546, -5.3665) (15.9214, -5.3331) (15.888, -5.3) (15.8545, -5.2672) (15.8208, -5.2346) (15.787, -5.2023) (15.753, -5.1703) (15.7188, -5.1386) (15.6846, -5.1071) (15.6501, -5.076) (15.6155, -5.0451) (15.5808, -5.0145) (15.5459, -4.9843) (15.5108, -4.9544) (15.4756, -4.9247) (15.4402, -4.8954) (15.4047, -4.8665) (15.369, -4.8378) (15.3332, -4.8094) (15.2972, -4.7814) (15.2611, -4.7538) (15.2247, -4.7265) (15.1882, -4.6996) (15.1516, -4.6731) (15.1147, -4.647) (15.0777, -4.6213) (15.0406, -4.5959) (15.0033, -4.5709) (14.9658, -4.5462) (14.9282, -4.522) (14.8904, -4.4982) (14.8523, -4.4751) (14.814, -4.4526) (14.7754, -4.4307) (14.7367, -4.4094) (14.6977, -4.3885) (14.6587, -4.3679) (14.6196, -4.3477) (14.5803, -4.3278) (14.5407, -4.3088) (14.5007, -4.2912) (14.4681, -4.2785) (14.4433, -4.27) (14.4267, -4.2648) (14.4183, -4.2623) knots -1 -1 -1 -1 -1 -1 -0.98571429 -0.97142857 -0.95714286 -0.94285714 -0.92857143 -0.91428571 -0.9 -0.88571429 -0.87142857 -0.85714286 -0.84285714 -0.82857143 -0.81428571 -0.8 -0.78571429 -0.77142857 -0.75714286 -0.74285714 -0.72857143 -0.71428571 -0.7 -0.68571429 -0.67142857 -0.65714286 -0.64285714 -0.62857143 -0.61428571 -0.6 -0.58571429 -0.57142857 -0.55714286 -0.54285714 -0.52857143 -0.51428571 -0.5 -0.48571429 -0.47142857 -0.45714286 -0.44285714 -0.42857143 -0.41428571 -0.4 -0.38571429 -0.37142857 -0.35714286 -0.34285714 -0.32857143 -0.31428571 -0.3 -0.28571429 -0.27142857 -0.25714286 -0.24285714 -0.22857143 -0.21428571 -0.2 -0.18571429 -0.17142857 -0.15714286 -0.14285714 -0.12857143 -0.11428571 -0.1 -0.08571429 -0.07142857 -0.05714286 -0.04285714 -0.02857143 -0.01428571 0 0 0 0 0 0
  line L15 (14.4183, -4.2623) -> (14.0508, -4.1537)
  arc A31 (13.3583, -2.9772) -> (14.0508, -4.1537) centre (14.3343, -3.1947) ccw
  arc A32 (13.3583, -2.9772) -> (13.4807, -2.3614) centre (0, 0) ccw
  arc A33 (14.5708, -1.5395) -> (13.4807, -2.3614) centre (14.4657, -2.534) ccw
  line L16 (14.5708, -1.5395) -> (14.9519, -1.5798)
  spline S16 degree 5 poles (14.9519, -1.5798) (14.9606, -1.5807) (14.978, -1.5823) (15.0041, -1.5839) (15.039, -1.5847) (15.0828, -1.5837) (15.1266, -1.5812) (15.1705, -1.578) (15.2144, -1.5742) (15.2583, -1.5701) (15.3023, -1.5657) (15.3463, -1.5609) (15.3903, -1.5554) (15.4343, -1.5493) (15.4783, -1.5425) (15.5224, -1.535) (15.5664, -1.527) (15.6104, -1.5186) (15.6545, -1.5097) (15.6985, -1.5005) (15.7425, -1.4909) (15.7866, -1.4808) (15.8306, -1.4704) (15.8746, -1.4595) (15.9186, -1.4482) (15.9626, -1.4365) (16.0065, -1.4244) (16.0505, -1.4119) (16.0944, -1.3991) (16.1383, -1.3859) (16.1822, -1.3724) (16.2261, -1.3585) (16.2699, -1.3443) (16.3137, -1.3297) (16.3575, -1.3147) (16.4013, -1.2995) (16.4451, -1.2839) (16.4888, -1.2679) (16.5324, -1.2517) (16.5761, -1.2351) (16.6197, -1.2182) (16.6633, -1.201) (16.7068, -1.1835) (16.7504, -1.1657) (16.7938, -1.1475) (16.8373, -1.1291) (16.8807, -1.1104) (16.924, -1.0913) (16.9674, -1.072) (17.0106, -1.0524) (17.0539, -1.0325) (17.0971, -1.0123) (17.1402, -0.9918) (17.1833, -0.9711) (17.2264, -0.95) (17.2694, -0.9287) (17.3123, -0.9071) (17.3552, -0.8852) (17.3981, -0.863) (17.4409, -0.8406) (17.4837, -0.8179) (17.5264, -0.795) (17.569, -0.7717) (17.6116, -0.7482) (17.6541, -0.7245) (17.6966, -0.7004) (17.7391, -0.6762) (17.7814, -0.6516) (17.8237, -0.6268) (17.866, -0.6018) (17.9082, -0.5765) (17.9419, -0.556) (17.9671, -0.5405) (17.9839, -0.5302) (17.9923, -0.525) knots 0 0 0 0 0 0 0.01428571 0.02857143 0.04285714 0.05714286 0.07142857 0.08571429 0.1 0.11428571 0.12857143 0.14285714 0.15714286 0.17142857 0.18571429 0.2 0.21428571 0.22857143 0.24285714 0.25714286 0.27142857 0.28571429 0.3 0.31428571 0.32857143 0.34285714 0.35714286 0.37142857 0.38571429 0.4 0.41428571 0.42857143 0.44285714 0.45714286 0.47142857 0.48571429 0.5 0.51428571 0.52857143 0.54285714 0.55714286 0.57142857 0.58571429 0.6 0.61428571 0.62857143 0.64285714 0.65714286 0.67142857 0.68571429 0.7 0.71428571 0.72857143 0.74285714 0.75714286 0.77142857 0.78571429 0.8 0.81428571 0.82857143 0.84285714 0.85714286 0.87142857 0.88571429 0.9 0.91428571 0.92857143 0.94285714 0.95714286 0.97142857 0.98571429 1 1 1 1 1 1
  arc A34 (17.9923, -0.525) -> (17.9923, 0.525) centre (0, 0) ccw
  spline S17 degree 5 poles (17.9923, 0.525) (17.9839, 0.5302) (17.9671, 0.5405) (17.9419, 0.556) (17.9082, 0.5765) (17.866, 0.6018) (17.8237, 0.6268) (17.7814, 0.6516) (17.7391, 0.6762) (17.6966, 0.7004) (17.6541, 0.7245) (17.6116, 0.7482) (17.569, 0.7717) (17.5264, 0.795) (17.4837, 0.8179) (17.4409, 0.8406) (17.3981, 0.863) (17.3552, 0.8852) (17.3123, 0.9071) (17.2694, 0.9287) (17.2264, 0.95) (17.1833, 0.9711) (17.1402, 0.9918) (17.0971, 1.0123) (17.0539, 1.0325) (17.0106, 1.0524) (16.9674, 1.072) (16.924, 1.0913) (16.8807, 1.1104) (16.8373, 1.1291) (16.7938, 1.1475) (16.7504, 1.1657) (16.7068, 1.1835) (16.6633, 1.201) (16.6197, 1.2182) (16.5761, 1.2351) (16.5324, 1.2517) (16.4888, 1.2679) (16.4451, 1.2839) (16.4013, 1.2995) (16.3575, 1.3147) (16.3137, 1.3297) (16.2699, 1.3443) (16.2261, 1.3585) (16.1822, 1.3724) (16.1383, 1.3859) (16.0944, 1.3991) (16.0505, 1.4119) (16.0065, 1.4244) (15.9626, 1.4365) (15.9186, 1.4482) (15.8746, 1.4595) (15.8306, 1.4704) (15.7866, 1.4808) (15.7425, 1.4909) (15.6985, 1.5005) (15.6545, 1.5097) (15.6104, 1.5186) (15.5664, 1.527) (15.5224, 1.535) (15.4783, 1.5425) (15.4343, 1.5493) (15.3903, 1.5554) (15.3463, 1.5609) (15.3023, 1.5657) (15.2583, 1.5701) (15.2144, 1.5742) (15.1705, 1.578) (15.1266, 1.5812) (15.0828, 1.5837) (15.039, 1.5847) (15.0041, 1.5839) (14.978, 1.5823) (14.9606, 1.5807) (14.9519, 1.5798) knots -1 -1 -1 -1 -1 -1 -0.98571429 -0.97142857 -0.95714286 -0.94285714 -0.92857143 -0.91428571 -0.9 -0.88571429 -0.87142857 -0.85714286 -0.84285714 -0.82857143 -0.81428571 -0.8 -0.78571429 -0.77142857 -0.75714286 -0.74285714 -0.72857143 -0.71428571 -0.7 -0.68571429 -0.67142857 -0.65714286 -0.64285714 -0.62857143 -0.61428571 -0.6 -0.58571429 -0.57142857 -0.55714286 -0.54285714 -0.52857143 -0.51428571 -0.5 -0.48571429 -0.47142857 -0.45714286 -0.44285714 -0.42857143 -0.41428571 -0.4 -0.38571429 -0.37142857 -0.35714286 -0.34285714 -0.32857143 -0.31428571 -0.3 -0.28571429 -0.27142857 -0.25714286 -0.24285714 -0.22857143 -0.21428571 -0.2 -0.18571429 -0.17142857 -0.15714286 -0.14285714 -0.12857143 -0.11428571 -0.1 -0.08571429 -0.07142857 -0.05714286 -0.04285714 -0.02857143 -0.01428571 0 0 0 0 0 0
  line L17 (14.9519, 1.5798) -> (14.5708, 1.5395)
  arc A35 (13.4807, 2.3614) -> (14.5708, 1.5395) centre (14.4657, 2.534) ccw
  arc A36 (13.4807, 2.3614) -> (13.3583, 2.9772) centre (0, 0) ccw
  arc A37 (14.0508, 4.1537) -> (13.3583, 2.9772) centre (14.3343, 3.1947) ccw
  line L18 (14.0508, 4.1537) -> (14.4183, 4.2623)
  spline S18 degree 5 poles (14.4183, 4.2623) (14.4267, 4.2648) (14.4433, 4.27) (14.4681, 4.2785) (14.5007, 4.2912) (14.5407, 4.3088) (14.5803, 4.3278) (14.6196, 4.3477) (14.6587, 4.3679) (14.6977, 4.3885) (14.7367, 4.4094) (14.7754, 4.4307) (14.814, 4.4526) (14.8523, 4.4751) (14.8904, 4.4982) (14.9282, 4.522) (14.9658, 4.5462) (15.0033, 4.5709) (15.0406, 4.5959) (15.0777, 4.6213) (15.1147, 4.647) (15.1516, 4.6731) (15.1882, 4.6996) (15.2247, 4.7265) (15.2611, 4.7538) (15.2972, 4.7814) (15.3332, 4.8094) (15.369, 4.8378) (15.4047, 4.8665) (15.4402, 4.8954) (15.4756, 4.9247) (15.5108, 4.9544) (15.5459, 4.9843) (15.5808, 5.0145) (15.6155, 5.0451) (15.6501, 5.076) (15.6846, 5.1071) (15.7188, 5.1386) (15.753, 5.1703) (15.787, 5.2023) (15.8208, 5.2346) (15.8545, 5.2672) (15.888, 5.3) (15.9214, 5.3331) (15.9546, 5.3665) (15.9877, 5.4002) (16.0206, 5.4341) (16.0534, 5.4683) (16.086, 5.5027) (16.1185, 5.5374) (16.1508, 5.5723) (16.183, 5.6075) (16.215, 5.6429) (16.2469, 5.6786) (16.2786, 5.7145) (16.3102, 5.7507) (16.3416, 5.7871) (16.3729, 5.8237) (16.404, 5.8606) (16.435, 5.8977) (16.4658, 5.935) (16.4965, 5.9726) (16.527, 6.0104) (16.5573, 6.0484) (16.5875, 6.0866) (16.6176, 6.1251) (16.6475, 6.1637) (16.6773, 6.2026) (16.7068, 6.2417) (16.7363, 6.2811) (16.7656, 6.3206) (16.7889, 6.3524) (16.8063, 6.3763) (16.8179, 6.3923) (16.8237, 6.4003) knots 0 0 0 0 0 0 0.01428571 0.02857143 0.04285714 0.05714286 0.07142857 0.08571429 0.1 0.11428571 0.12857143 0.14285714 0.15714286 0.17142857 0.18571429 0.2 0.21428571 0.22857143 0.24285714 0.25714286 0.27142857 0.28571429 0.3 0.31428571 0.32857143 0.34285714 0.35714286 0.37142857 0.38571429 0.4 0.41428571 0.42857143 0.44285714 0.45714286 0.47142857 0.48571429 0.5 0.51428571 0.52857143 0.54285714 0.55714286 0.57142857 0.58571429 0.6 0.61428571 0.62857143 0.64285714 0.65714286 0.67142857 0.68571429 0.7 0.71428571 0.72857143 0.74285714 0.75714286 0.77142857 0.78571429 0.8 0.81428571 0.82857143 0.84285714 0.85714286 0.87142857 0.88571429 0.9 0.91428571 0.92857143 0.94285714 0.95714286 0.97142857 0.98571429 1 1 1 1 1 1
  arc A38 (16.8237, 6.4003) -> (16.4218, 7.3704) centre (0, 0) ccw
  spline S19 degree 5 poles (16.4218, 7.3704) (16.4121, 7.372) (16.3926, 7.3751) (16.3633, 7.3797) (16.3244, 7.3857) (16.2757, 7.393) (16.2271, 7.4) (16.1785, 7.4067) (16.13, 7.4131) (16.0815, 7.4193) (16.0331, 7.4253) (15.9847, 7.4309) (15.9363, 7.4364) (15.888, 7.4415) (15.8398, 7.4464) (15.7916, 7.451) (15.7435, 7.4553) (15.6954, 7.4594) (15.6474, 7.4632) (15.5994, 7.4667) (15.5515, 7.4699) (15.5037, 7.4729) (15.4559, 7.4756) (15.4082, 7.478) (15.3606, 7.4801) (15.313, 7.482) (15.2655, 7.4835) (15.2181, 7.4848) (15.1708, 7.4858) (15.1235, 7.4865) (15.0763, 7.4869) (15.0292, 7.487) (14.9822, 7.4868) (14.9353, 7.4864) (14.8884, 7.4856) (14.8417, 7.4845) (14.795, 7.4831) (14.7484, 7.4814) (14.7019, 7.4794) (14.6555, 7.4771) (14.6093, 7.4744) (14.5631, 7.4715) (14.517, 7.4682) (14.4711, 7.4645) (14.4252, 7.4606) (14.3795, 7.4563) (14.3339, 7.4517) (14.2884, 7.4467) (14.243, 7.4414) (14.1977, 7.4358) (14.1526, 7.4298) (14.1077, 7.4234) (14.0628, 7.4166) (14.0182, 7.4094) (13.9737, 7.4018) (13.9293, 7.3938) (13.8851, 7.3855) (13.841, 7.3768) (13.7971, 7.3678) (13.7534, 7.3583) (13.7098, 7.3484) (13.6665, 7.3378) (13.6235, 7.3266) (13.5808, 7.3148) (13.5383, 7.3025) (13.496, 7.2897) (13.4539, 7.2767) (13.4118, 7.2633) (13.3701, 7.2496) (13.3286, 7.235) (13.2878, 7.2192) (13.2559, 7.2052) (13.2323, 7.1937) (13.2168, 7.1855) (13.2092, 7.1813) knots -1 -1 -1 -1 -1 -1 -0.98571429 -0.97142857 -0.95714286 -0.94285714 -0.92857143 -0.91428571 -0.9 -0.88571429 -0.87142857 -0.85714286 -0.84285714 -0.82857143 -0.81428571 -0.8 -0.78571429 -0.77142857 -0.75714286 -0.74285714 -0.72857143 -0.71428571 -0.7 -0.68571429 -0.67142857 -0.65714286 -0.64285714 -0.62857143 -0.61428571 -0.6 -0.58571429 -0.57142857 -0.55714286 -0.54285714 -0.52857143 -0.51428571 -0.5 -0.48571429 -0.47142857 -0.45714286 -0.44285714 -0.42857143 -0.41428571 -0.4 -0.38571429 -0.37142857 -0.35714286 -0.34285714 -0.32857143 -0.31428571 -0.3 -0.28571429 -0.27142857 -0.25714286 -0.24285714 -0.22857143 -0.21428571 -0.2 -0.18571429 -0.17142857 -0.15714286 -0.14285714 -0.12857143 -0.11428571 -0.1 -0.08571429 -0.07142857 -0.05714286 -0.04285714 -0.02857143 -0.01428571 0 0 0 0 0 0
  line L19 (13.2092, 7.1813) -> (12.8725, 6.9983)
  arc A39 (11.5509, 7.3405) -> (12.8725, 6.9983) centre (12.3949, 7.8769) ccw
  arc A40 (11.5509, 7.3405) -> (11.2021, 7.8625) centre (0, 0) ccw
  arc A41 (11.3917, 9.2145) -> (11.2021, 7.8625) centre (12.0206, 8.437) ccw
  line L20 (11.3917, 9.2145) -> (11.6896, 9.4555)